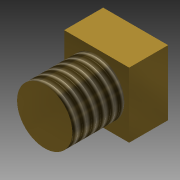
# Autodesk Inventor part: PSI Gauge Screw 1764
Saved by Autodesk Inventor 2011 (Build 150239000, 239)
## iProperties
Created: 2010-02-12
Part Number: PSI Gauge Screw 1764
Document SubType Name: Modeling
Designer: jgehrig
Density: 1 g/cm^3
Author: jgehrig
Autodesk Inventor part; units mm, degrees
ref_plane "YZ Plane" through (0, 0, 0) normal (1, 0, 0) x (0, 1, 0)
ref_plane "XZ Plane" through (0, 0, 0) normal (0, 1, 0) x (-1, 0, 0)
ref_plane "XY Plane" through (0, 0, 0) normal (0, 0, 1) x (1, 0, 0)
sketch "Sketch1" plane through (0, 0, 0) normal (0, 0, 1) x (1, 0, 0)
  line L0 (-10.3865, 10.7488) -> (2.3135, 10.7488)
  line L1 (2.3135, 10.7488) -> (2.3135, -1.9512)
  line L2 (2.3135, -1.9512) -> (-10.3865, -1.9512)
  line L3 (-10.3865, -1.9512) -> (-10.3865, 10.7488)
  point P0 (0, 0)
  dimension "d0" = 12.7
  dimension "d1" = 12.7
  constraints: 8 end point, 2 parallel, 1 horizontal, 1 perpendicular
  measures "d0" distance of L0.start L0.end
  measures "d1" distance of L2.end L0.start
extrude "Extrusion1" add sketch "Sketch1" along normal blind 7.62
sketch "Sketch2" plane through (0, 0, 7.62) normal (0, 0, 1) x (1, 0, 0)
  circle A0 centre (-4.0365, 4.3988) radius 5.3975
  point P0 (0, 0)
  dimension "d4" = 10.795
  constraints: 1 centre point
  measures "d4" diameter of A0
extrude "Extrusion2" add sketch "Sketch2" along normal blind 10.16
thread "Thread1" size "7/16-14 UNC" class "2A" standard "ANSI Unified Screw Threads" full length
body "Solid1"
